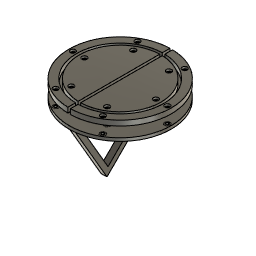
taiko v7 (Autodesk Fusion 360 design; units mm, degrees)
Autodesk Fusion 360 part; units mm, degrees
sketch "Sketch3" plane through (0, 0, 0) normal (0, 0, 1) x (1, 0, 0)
  circle A0 centre (0, 0) radius 100
  dimension "d6" = 200
  constraint coincident A0.centre origin
  measures "d6" diameter of A0
extrude "Extrude2" add sketch "Sketch3" along normal blind 5 makes body 1
sketch "Sketch4" plane through (0, 0, 5) normal (0, 0, 1) x (-1, 0, 0)
  circle A0 centre (0, 0) radius 100
  circle A1 centre (0, 0) radius 80
  circle A2 centre (0, 0) radius 85
  line L0 (100, -100) -> (-100, -100)
  line L1 (-100, -100) -> (-100, 100)
  line L2 (-100, 100) -> (100, 100)
  line L3 (100, 100) -> (100, -100)
  line L4 (0, -100) -> (0, 100)
  line L5 (2.5, -100) -> (2.5, 99.9687)
  line L6 (-2.5, -99.9687) -> (-2.5, 99.9687)
  point P0 (-70, 0)
  dimension "d9" = 160
  dimension "d13" = 5
  dimension "d14" = 200
  dimension "d15" = 200
  dimension "d16" = 2.5
  dimension "d17" = 100
  dimension "d18" = 2.5
  constraint coincident A0.centre A1.centre
  constraint horizontal L0
  constraint vertical L1
  constraint horizontal L2
  constraint vertical L3
  constraint midpoint L0 L4.start
  constraint midpoint L2 L4.end
  constraint coincident L0 L5.start
  constraint coincident A0 L5.end
  constraint perpendicular L2 L5
  constraint coincident A0 L6.start
  constraint coincident A0 L6.end
  constraint perpendicular L2 L6
  measures "d9" diameter of A1
  measures "d13" distance of A1 A2
  measures "d14" distance of L0.start L0.end
  measures "d15" distance of L0.start L2.end
  measures "d16" distance of L4 L5
  measures "d17" distance of A0.centre L3
  measures "d18" distance of L4 L6
extrude "Extrude3" add sketch "Sketch4" along normal blind 10 separate body contours A0 A2 L5 | A0 A2 L6 | A1 L5 | A1 L6 makes body 2 at (-7.379, 94.4842, 15) makes body 3 at (-34.332, -9.5574, 5) makes body 4 at (7.379, 94.4842, 5) makes body 5 at (26.5618, 9.5574, 5)
sketch "Sketch5" plane through (0, 0, 0) normal (0, 0, 1) x (1, 0, 0)
sketch "Sketch6" plane through (0, 0, 15) normal (0, 0, 1) x (-1, 0, 0)
  arc A0 (-2.5, 79.9609) -> (-2.5, -79.9609) centre (0, 0) ccw
  line L0 (-2.5, -79.9609) -> (-2.5, 79.9609)
  point P0 (-70, 0)
hole "Hole1" at (70, 0, 15) direction (0, 0, -1) diameter 6 depth 40 tip angle 118 counterbore diameter 10 counterbore depth 4 bodies 1 5
pattern_circular "C-Pattern1" count 6 over 360 about axis through (0, 0, 1.75) along (0, 0, 1) of "Hole1"
sketch "Sketch7" plane through (0, 0, 15) normal (0, 0, 1) x (-1, 0, 0)
  arc A0 (2.5, -79.9609) -> (2.5, 79.9609) centre (0, 0) ccw
  line L0 (2.5, 79.9609) -> (2.5, -79.9609)
  point P0 (70, 0)
hole "Hole2" at (-70, 0, 15) direction (0, 0, -1) diameter 6 depth 40 tip angle 118 counterbore diameter 10 counterbore depth 4 bodies 3
pattern_circular "C-Pattern2" count 6 over 360 about axis through (0, 0, 1.75) along (0, 0, 1) of "Hole2"
sketch "Sketch8" plane through (0, 0, 15) normal (0, 0, 1) x (-1, 0, 0)
  arc A0 (2.5, -99.9687) -> (2.5, 99.9687) centre (0, 0) ccw
  line L0 (2.5, 99.9687) -> (2.5, 84.9632)
  arc A1 (2.5, -84.9632) -> (2.5, 84.9632) centre (0, 0) ccw
  line L1 (2.5, -84.9632) -> (2.5, -99.9687)
  point P0 (92.5, 0)
  dimension "d35" = 92.5
  measures "d35" distance of A0.centre P0
hole "Hole3" at (-92.5, 0, 15) direction (0, 0, -1) diameter 6 depth 40 tip angle 118 counterbore diameter 10 counterbore depth 4 bodies 1 2
pattern_circular "C-Pattern3" count 6 over 360 about axis through (0, 0, 1.75) along (0, 0, 1) of "Hole3"
sketch "Sketch9" plane through (0, 0, 15) normal (0, 0, 1) x (-1, 0, 0)
  line L0 (-2.5, 84.9632) -> (-2.5, 99.9687)
  arc A0 (-2.5, 99.9687) -> (-2.5, -99.9687) centre (0, 0) ccw
  line L1 (-2.5, -99.9687) -> (-2.5, -84.9632)
  arc A1 (-2.5, 84.9632) -> (-2.5, -84.9632) centre (0, 0) ccw
  point P0 (-92.5, 0)
  dimension "d43" = 92.5
  measures "d43" distance of A0.centre P0
hole "Hole4" at (92.5, 0, 15) direction (0, 0, -1) diameter 6 depth 40 tip angle 118 counterbore diameter 10 counterbore depth 4 bodies 4
pattern_circular "C-Pattern4" count 6 over 360 about axis through (0, 0, 1.75) along (0, 0, 1) of "Hole4"
move_body "Move1" bodies 2 3 4 5 to x (1, 0, 0) y (0, 1, 0) z (0, 0, 1) at (0, 0, 20)
extrude "Extrude4" add 1 faces at (-11.0889, -19.3911, 0) along direction (0, 0, -1) blind 1 on bodies 1 bodies 1
sketch "Sketch10" plane through (0, 0, -1) normal (0, 0, -1) x (1, 0, 0)
  circle A0 centre (-46.25, -80.1073) radius 3
  circle A1 centre (46.25, -80.1073) radius 3
  circle A2 centre (92.5, 0) radius 3
  circle A3 centre (46.25, 80.1073) radius 3
  circle A4 centre (-46.25, 80.1073) radius 3
  circle A5 centre (-92.5, 0) radius 3
  circle A6 centre (35, 60.6218) radius 3
  circle A7 centre (-35, 60.6218) radius 3
  circle A8 centre (-70, 0) radius 3
  circle A9 centre (-35, -60.6218) radius 3
  circle A10 centre (35, -60.6218) radius 3
  circle A11 centre (70, 0) radius 3
  circle A12 centre (0, 0) radius 100
  line L0 (-95.3868, 5) -> (-98.2735, 0)
  line L1 (-98.2735, 0) -> (-95.3868, -5)
  line L2 (-95.3868, -5) -> (-89.6132, -5)
  line L3 (-89.6132, -5) -> (-86.7265, 0)
  line L4 (-86.7265, 0) -> (-89.6132, 5)
  line L5 (-89.6132, 5) -> (-95.3868, 5)
  line L6 (-72.8868, 5) -> (-75.7735, 0)
  line L7 (-75.7735, 0) -> (-72.8868, -5)
  line L8 (-72.8868, -5) -> (-67.1132, -5)
  line L9 (-67.1132, -5) -> (-64.2265, 0)
  line L10 (-64.2265, 0) -> (-67.1132, 5)
  line L11 (-67.1132, 5) -> (-72.8868, 5)
  point P0 (-92.5, 0)
  point P1 (-70, 0)
  dimension "d53" = 5
  dimension "d58" = 5
  constraint coincident P0 A5.centre
  constraint coincident P1 A8.centre
  measures "d53" distance of P0 L5
  measures "d58" distance of P1 L11
extrude "Extrude5" cut sketch "Sketch10" against normal blind 5 contours L0 L1 L2 L3 L4 L5 bodies 1
pattern_circular "C-Pattern5" count 6 over 360 about axis through (0, 0, 1.75) along (0, 0, 1) of "Extrude5"
extrude "Extrude6" cut sketch "Sketch10" against normal blind 5 contours L6 L7 L8 L9 L10 L11 bodies 1
pattern_circular "C-Pattern6" count 6 over 360 about axis through (0, 0, 1.75) along (0, 0, 1) of "Extrude6"
sketch "Sketch11" plane through (0, 0, -1) normal (0, 0, -1) x (1, 0, 0)
  line L0 (-37.8868, -65.6218) -> (-40.7735, -60.6218)
  line L1 (-40.7735, -60.6218) -> (-37.8868, -55.6218)
  line L2 (-37.8868, -55.6218) -> (-32.1132, -55.6218)
  line L3 (-32.1132, -55.6218) -> (-29.2265, -60.6218)
  line L4 (-29.2265, -60.6218) -> (-32.1132, -65.6218)
  line L5 (-32.1132, -65.6218) -> (-37.8868, -65.6218)
  line L6 (37.8868, -65.6218) -> (32.1132, -65.6218)
  line L7 (32.1132, -65.6218) -> (29.2265, -60.6218)
  line L8 (29.2265, -60.6218) -> (32.1132, -55.6218)
  line L9 (32.1132, -55.6218) -> (37.8868, -55.6218)
  line L10 (37.8868, -55.6218) -> (40.7735, -60.6218)
  line L11 (40.7735, -60.6218) -> (37.8868, -65.6218)
  line L12 (75.7735, 0) -> (72.8868, -5)
  line L13 (72.8868, -5) -> (67.1132, -5)
  line L14 (67.1132, -5) -> (64.2265, 0)
  line L15 (64.2265, 0) -> (67.1132, 5)
  line L16 (67.1132, 5) -> (72.8868, 5)
  line L17 (72.8868, 5) -> (75.7735, 0)
  line L18 (37.8868, 65.6218) -> (40.7735, 60.6218)
  line L19 (40.7735, 60.6218) -> (37.8868, 55.6218)
  line L20 (37.8868, 55.6218) -> (32.1132, 55.6218)
  line L21 (32.1132, 55.6218) -> (29.2265, 60.6218)
  line L22 (29.2265, 60.6218) -> (32.1132, 65.6218)
  line L23 (32.1132, 65.6218) -> (37.8868, 65.6218)
  line L24 (-37.8868, 65.6218) -> (-32.1132, 65.6218)
  line L25 (-32.1132, 65.6218) -> (-29.2265, 60.6218)
  line L26 (-29.2265, 60.6218) -> (-32.1132, 55.6218)
  line L27 (-32.1132, 55.6218) -> (-37.8868, 55.6218)
  line L28 (-37.8868, 55.6218) -> (-40.7735, 60.6218)
  line L29 (-40.7735, 60.6218) -> (-37.8868, 65.6218)
  line L30 (-75.7735, 0) -> (-72.8868, 5)
  line L31 (-72.8868, 5) -> (-67.1132, 5)
  line L32 (-67.1132, 5) -> (-64.2265, 0)
  line L33 (-64.2265, 0) -> (-67.1132, -5)
  line L34 (-67.1132, -5) -> (-72.8868, -5)
  line L35 (-72.8868, -5) -> (-75.7735, 0)
  line L36 (-49.1368, -85.1073) -> (-52.0235, -80.1073)
  line L37 (-52.0235, -80.1073) -> (-49.1368, -75.1073)
  line L38 (-49.1368, -75.1073) -> (-43.3632, -75.1073)
  line L39 (-43.3632, -75.1073) -> (-40.4765, -80.1073)
  line L40 (-40.4765, -80.1073) -> (-43.3632, -85.1073)
  line L41 (-43.3632, -85.1073) -> (-49.1368, -85.1073)
  line L42 (49.1368, -85.1073) -> (43.3632, -85.1073)
  line L43 (43.3632, -85.1073) -> (40.4765, -80.1073)
  line L44 (40.4765, -80.1073) -> (43.3632, -75.1073)
  line L45 (43.3632, -75.1073) -> (49.1368, -75.1073)
  line L46 (49.1368, -75.1073) -> (52.0235, -80.1073)
  line L47 (52.0235, -80.1073) -> (49.1368, -85.1073)
  line L48 (98.2735, 0) -> (95.3868, -5)
  line L49 (95.3868, -5) -> (89.6132, -5)
  line L50 (89.6132, -5) -> (86.7265, 0)
  line L51 (86.7265, 0) -> (89.6132, 5)
  line L52 (89.6132, 5) -> (95.3868, 5)
  line L53 (95.3868, 5) -> (98.2735, 0)
  line L54 (49.1368, 85.1073) -> (52.0235, 80.1073)
  line L55 (52.0235, 80.1073) -> (49.1368, 75.1073)
  line L56 (49.1368, 75.1073) -> (43.3632, 75.1073)
  line L57 (43.3632, 75.1073) -> (40.4765, 80.1073)
  line L58 (40.4765, 80.1073) -> (43.3632, 85.1073)
  line L59 (43.3632, 85.1073) -> (49.1368, 85.1073)
  line L60 (-49.1368, 85.1073) -> (-43.3632, 85.1073)
  line L61 (-43.3632, 85.1073) -> (-40.4765, 80.1073)
  line L62 (-40.4765, 80.1073) -> (-43.3632, 75.1073)
  line L63 (-43.3632, 75.1073) -> (-49.1368, 75.1073)
  line L64 (-49.1368, 75.1073) -> (-52.0235, 80.1073)
  line L65 (-52.0235, 80.1073) -> (-49.1368, 85.1073)
  line L66 (-98.2735, 0) -> (-95.3868, 5)
  line L67 (-95.3868, 5) -> (-89.6132, 5)
  line L68 (-89.6132, 5) -> (-86.7265, 0)
  line L69 (-86.7265, 0) -> (-89.6132, -5)
  line L70 (-89.6132, -5) -> (-95.3868, -5)
  line L71 (-95.3868, -5) -> (-98.2735, 0)
  circle A0 centre (0, 0) radius 100
  line L72 (-40.7735, 70.6218) -> (-29.2265, 70.6218)
  line L73 (-29.2265, 70.6218) -> (-29.2265, -70.6218)
  line L74 (-29.2265, -70.6218) -> (-40.7735, -70.6218)
  line L75 (-40.7735, -70.6218) -> (-40.7735, 70.6218)
  dimension "d63" = 5
  dimension "d64" = 5
  constraint horizontal L72
  constraint vertical L73
  constraint horizontal L74
  constraint vertical L75
  measures "d63" distance of L24 L72
  measures "d64" distance of L5 L74
extrude "Extrude7" add sketch "Sketch11" along normal blind 10 separate body contours L0 L4 L5 L73 L74 L75 | L0 L1 L2 L3 L4 L5 | L1 L2 L3 L26 L27 L28 L73 L75 | L24 L25 L26 L27 L28 L29 | L24 L25 L29 L72 L73 L75 makes body 6
move_body "Move2" bodies 6 to x (1, 0, 0) y (0, 1, 0) z (0, 0, 1) at (0, 0, -10)
extrude "Extrude9" add 1 faces at (-33.0755, 70.6218, -14.3333) along direction (0, 1, 0) blind 60 on bodies 6 bodies 6
sketch "Sketch12" plane through (0, 0, -21) normal (0, 0, -1) x (1, 0, 0)
  line L0 (-29.2265, -130.6218) -> (-29.2265, 70.6218)
  line L1 (-29.2265, 70.6218) -> (-40.7735, 70.6218)
  line L2 (-40.7735, 70.6218) -> (-40.7735, -130.6218)
  line L3 (-40.7735, -130.6218) -> (-29.2265, -130.6218)
  circle A0 centre (-35, -60.6218) radius 3
  line L4 (-40.7735, -130.6218) -> (-29.2265, -130.6218)
  line L5 (-40.7735, -130.6218) -> (-40.7735, 70.6218)
  line L6 (-40.7735, 70.6218) -> (-29.2265, 70.6218)
  line L7 (-29.2265, 70.6218) -> (-29.2265, -130.6218)
  point P0 (-35, 60.6218)
hole "Hole5" at (-35, 60.6218, -21) direction (0, 0, 1) diameter 6 depth 10 tip angle 118 bodies 6
sketch "Sketch13" plane through (-40.7735, 0, 0) normal (-1, 0, 0) x (0, -1, 0)
  line L0 (70.6218, -11) -> (-130.6218, -11)
  line L1 (-130.6218, -11) -> (-130.6218, -21)
  line L2 (-130.6218, -21) -> (70.6218, -21)
  line L3 (70.6218, -21) -> (70.6218, -11)
  line L4 (-130.6218, -21) -> (39.3782, -21) construction
  constraint horizontal L4
  constraint coincident L1.end L2.start
sketch "Sketch14" plane through (-29.2265, 0, 0) normal (1, 0, 0) x (0, 1, 0)
  line L0 (130.6218, -11) -> (-70.6218, -11)
  line L1 (-70.6218, -11) -> (-70.6218, -21)
  line L2 (-70.6218, -21) -> (130.6218, -21)
  line L3 (130.6218, -21) -> (3.3426, -148.2792)
  line L4 (-70.6218, -21) -> (3.3426, -148.2792)
  line L5 (116.4796, -21) -> (-1.8552, -139.3348)
  line L6 (-59.0559, -21) -> (10.6576, -140.9642)
  line L7 (130.6218, -21) -> (-39.3782, -21)
  dimension "d91" = 180
  dimension "d93" = 10
  dimension "d94" = 10
  dimension "d95" = 45
  constraint coincident L2.end L3.start
  constraint coincident L1.end L2.start
  constraint coincident L2 L5.start
  constraint coincident L4 L5.end
  constraint coincident L2 L6.start
  constraint coincident L3 L6.end
  constraint parallel L4 L6
  measures "d91" distance of L2.end L3.end
  measures "d93" distance of L3 L5
  measures "d94" distance of L4 L6
  measures "d95" angle of L5 L7
extrude "Extrude11" add sketch "Sketch14" against normal blind 11.547 contours L2 L4 L5 L6 | L3 L4 L5 L6 | L2 L3 L5 L6 L7 bodies 6
hole "Hole8" at (-35, -60.6218, -1) direction (0, 0, -1) diameter 6 depth 44 tip angle 118 bodies 6
move_body "Move3" [suppressed]
move_body "Move4" [suppressed]
hole "Hole7" [suppressed]
equation "d35 = 100 mm - 7.5 mm"
equation "d43 = 100 mm - 7.5 mm"
named bodies: "backplate", "left ka", "left don", "right ka", "right don", "stand1"
